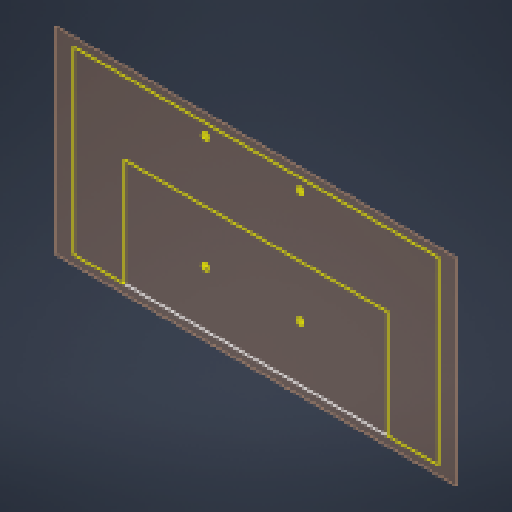
# Autodesk Inventor part: daiza
Saved by Autodesk Inventor 2026.1 (Build 301233020, 233B)
## iProperties
Created: 2026-03-17
Part Number: daiza
Material: 一般
Document SubType Name: Modeling
Designer: kamada
Density: 1 g/cm^3
Appearance: 既定
Author: kamada
Autodesk Inventor part; units mm, degrees
ref_plane "YZ Plane" through (0, 0, 0) normal (1, 0, 0) x (0, 1, 0)
ref_plane "XZ Plane" through (0, 0, 0) normal (0, 1, 0) x (-1, 0, 0)
ref_plane "XY Plane" through (0, 0, 0) normal (0, 0, 1) x (1, 0, 0)
ref_plane "作業平面1" through (0, 0, 0) normal (0, 0, 1) x (1, 0, 0)
sketch "スケッチ1" plane through (0, 0, 0) normal (0, 0, 1) x (1, 0, 0)
  circle A0 centre (49.1513, 36.4901) radius 0.75 projected
  circle A1 centre (49.1513, 11.9901) radius 0.75 projected
  circle A2 centre (28.6513, 11.9901) radius 0.75 projected
  circle A3 centre (28.6513, 36.4901) radius 0.75 projected
  line L0 (11.0939, 0) -> (11.0939, 23.2829) projected
  line L1 (11.0939, 23.2829) -> (68.0338, 23.2829) projected
  line L2 (68.0338, 23.2829) -> (68.0338, 0) projected
  line L3 (68.0338, 0) -> (79.1277, 0) projected
  line L4 (79.1277, 0) -> (79.1277, 38.98) projected
  line L5 (0, 38.98) -> (79.1277, 38.98) projected
  line L6 (0, 0) -> (0, 38.98) projected
  line L7 (0, 0) -> (11.0939, 0) projected
  line L8 (68.0338, 0) -> (11.0939, 0)
  constraints: 2 end point, 1 collinear
ref_plane "作業平面2" through (53.1084, 38.98, 5) normal (0, 1, 0) x (-1, 0, 0)
sketch "スケッチ2" plane through (53.1084, 38.98, 5) normal (0, 1, 0) x (-1, 0, 0)
  line L0 (0, 0) -> (27.0868, 0) projected
  line L1 (27.0868, 0) -> (27.0868, 3) projected
  line L2 (0, 3) -> (27.0868, 3) projected
  line L3 (0, 0) -> (0, 3) projected
  line L4 (53.1084, -5) -> (-26.0192, -5) projected
  line L5 (27.0868, 0) -> (53.1084, -5)
  line L6 (0, 0) -> (-26.0192, -5)
  line L7 (-14.9983, -5) -> (42.0865, -5)
  line L8 (42.0865, -5) -> (42.0865, -2.8822)
  line L9 (42.0865, -2.8822) -> (-14.9983, -2.8822)
  line L10 (-14.9983, -2.8822) -> (-14.9983, -5)
  point P0 (42.0865, -5)
  constraints: 12 end point, 3 point on line, 2 parallel, 1 horizontal, 1 perpendicular
ref_plane "作業平面3" through (-29.3223, 0, -100) normal (0, 1, 0) x (0, 0, 1)
extrude "押し出し1" add sketch "スケッチ2" against normal up to surface (38.98 mm away) contours L0 L5 L9 L6 | L9 L8 L4 L10
sketch "スケッチ3" plane through (68.1068, 38.98, 2.1178) normal (1, 0, 0) x (0, 0, -1)
  line L0 (2.1178, -38.98) -> (0, -38.98) projected
  line L1 (2.1178, 0) -> (2.1178, -38.98) projected
  line L2 (0, 0) -> (2.1178, 0) projected
  line L3 (0, 0) -> (0, -38.98) projected
  point P0 (2.1178, -38.98)
extrude "押し出し2" add sketch "スケッチ3" along normal blind 10
sketch "スケッチ4" plane through (11.0219, 38.98, 0) normal (-1, 0, 0) x (0, 0, 1)
  line L0 (2.1178, -38.98) -> (0, -38.98) projected
  line L1 (2.1178, 0) -> (2.1178, -38.98) projected
  line L2 (0, 0) -> (2.1178, 0) projected
  line L3 (0, 0) -> (0, -38.98) projected
  point P0 (0, -38.98)
extrude "押し出し3" add sketch "スケッチ4" along normal blind 10
